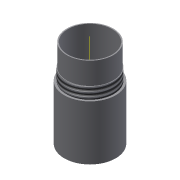
# Autodesk Inventor part: Vacuum Cylinder
Saved by Autodesk Inventor 2015 (Build 190159000, 159)
## iProperties
Created: 2014-07-08
Part Number: Vacuum Cylinder
Material: Generic
Document SubType Name: Modeling
Designer: I Rabey
Density: 1 g/cm^3
Appearance: Default
Author: I Rabey
Autodesk Inventor part; units mm, degrees
sketch "Sketch1" plane through (0, 0, 0) normal (0, 1, 0) x (-1, 0, 0)
  circle A0 centre (0, 0) radius 27.75
  circle A1 centre (0, 0) radius 32.25
  dimension "d0" = 55.5
  dimension "d1" = 64.5
  constraints: 2 centre point, 2 coincident
  measures "d0" diameter of A0
  measures "d1" diameter of A1
extrude "Extrusion1" add sketch "Sketch1" along normal blind 110.6
ref_plane "Work Plane1" through (0, 7.749, 0) normal (0, 1, 0) x (-1, 0, 0)
ref_plane "Work Plane2" through (0, 16.1, 0) normal (0, 1, 0) x (-1, 0, 0)
ref_plane "Work Plane3" through (0, 113.3, 0) normal (0, 1, 0) x (-1, 0, 0)
sketch "Sketch17" plane through (0, 110.6, 0) normal (0, 1, 0) x (1, 0, 0)
  circle A0 centre (0, 0) radius 29.75
  circle A1 centre (0, 0) radius 32.25
  dimension "d109" = 59.5
  constraints: 2 centre point, 2 coincident
  measures "d109" diameter of A0
extrude "Extrusion8" cut sketch "Sketch17" against normal blind 42
thread "Thread7" size "M60x5.5" class "6g" standard "ANSI Metric M Profile" full length
sketch "Sketch18" plane through (0, 110.6, 0) normal (0, 1, 0) x (1, 0, 0)
  circle A0 centre (0, 0) radius 32.1723
  circle A1 centre (0, 0) radius 29.1
  dimension "d114" = 58.2
  constraints: 2 centre point, 2 coincident
  measures "d114" diameter of A1
extrude "Extrusion9" cut sketch "Sketch18" against normal blind 27.5
body "Solid1"
